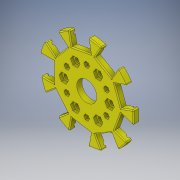
# Autodesk Inventor part: Frame
Saved by Autodesk Inventor 2016 (Build 200138000, 138)
## iProperties
Created: 2016-12-01
Part Number: Frame
Material: Generic
Document SubType Name: Modeling
Designer: Evan Phil George
Density: 1 g/cm^3
Appearance: Default
Author: Evan Phil George
Autodesk Inventor part; units mm, degrees
ref_plane "YZ Plane" through (0, 0, 0) normal (1, 0, 0) x (0, 1, 0)
ref_plane "XZ Plane" through (0, 0, 0) normal (0, 1, 0) x (-1, 0, 0)
ref_plane "XY Plane" through (0, 0, 0) normal (0, 0, 1) x (1, 0, 0)
sketch "Sketch1" plane through (0, 0, 0) normal (0, 0, 1) x (1, 0, 0)
  line L0 (0, 0) -> (49, 0)
  line L1 (0, 0) -> (-44.35, 0)
  line L2 (-44.35, 0) -> (-44.35, 10)
  line L3 (-44.35, 0) -> (-44.35, -10)
  line L4 (-44.35, 10) -> (-47.9687, 10)
  line L5 (-44.35, -10) -> (-47.9687, -10)
  line L6 (-44.35, 10) -> (-34.35, 10)
  line L7 (-34.35, 10) -> (-34.35, -10)
  line L8 (-34.35, -10) -> (-44.35, -10)
  line L9 (0, 0) -> (41.6754, 15.1686)
  line L10 (0, 0) -> (44.35, 0) construction
  line L11 (41.6754, 15.1686) -> (38.2552, 24.5655)
  line L12 (41.6754, 15.1686) -> (45.0956, 5.7717)
  line L13 (0, 0) -> (22.175, 38.4082)
  line L14 (0, 0) -> (44.35, 0) construction
  line L15 (22.175, 38.4082) -> (30.8353, 33.4082)
  line L16 (22.175, 38.4082) -> (13.5147, 43.4082)
  line L17 (0, 0) -> (-7.7013, 43.6762)
  line L18 (0, 0) -> (44.35, 0) construction
  line L19 (-7.7013, 43.6762) -> (2.1468, 45.4127)
  line L20 (-7.7013, 43.6762) -> (-17.5494, 41.9397)
  line L21 (0, 0) -> (-33.9741, 28.5076)
  line L22 (0, 0) -> (44.35, 0) construction
  line L23 (-33.9741, 28.5076) -> (-27.5462, 36.1681)
  line L24 (-33.9741, 28.5076) -> (-40.4019, 20.8472)
  line L25 (0, 0) -> (41.6754, -15.1686)
  line L26 (0, 0) -> (44.35, 0) construction
  line L27 (41.6754, -15.1686) -> (45.0956, -5.7717)
  line L28 (41.6754, -15.1686) -> (38.2552, -24.5655)
  line L29 (0, 0) -> (22.175, -38.4082)
  line L30 (0, 0) -> (44.35, 0) construction
  line L31 (22.175, -38.4082) -> (30.8353, -33.4082)
  line L32 (22.175, -38.4082) -> (13.5147, -43.4082)
  line L33 (0, 0) -> (-7.7013, -43.6762)
  line L34 (0, 0) -> (44.35, 0) construction
  line L35 (-7.7013, -43.6762) -> (2.1468, -45.4127)
  line L36 (-7.7013, -43.6762) -> (-17.5494, -41.9397)
  line L37 (0, 0) -> (-33.9741, -28.5076)
  line L38 (0, 0) -> (44.35, 0) construction
  line L39 (-33.9741, -28.5076) -> (-27.5462, -36.1681)
  line L40 (-33.9741, -28.5076) -> (-40.4019, -20.8472)
  line L41 (-27.5462, 36.1681) -> (-30.3183, 38.4942)
  line L42 (-40.4019, 20.8472) -> (-43.1741, 23.1733)
  line L43 (-27.5462, 36.1681) -> (-19.8858, 29.7402)
  line L44 (-40.4019, 20.8472) -> (-32.7415, 14.4193)
  line L45 (-17.5494, 41.9397) -> (-18.1778, 45.5035)
  line L46 (2.1468, 45.4127) -> (1.5184, 48.9765)
  line L47 (2.1468, 45.4127) -> (3.8833, 35.5646)
  line L48 (-17.5494, 41.9397) -> (-15.8129, 32.0917)
  line L49 (30.8353, 33.4082) -> (32.6446, 36.5421)
  line L50 (30.8353, 33.4082) -> (25.8353, 24.748)
  line L51 (13.5147, 43.4082) -> (15.3241, 46.5421)
  line L52 (13.5147, 43.4082) -> (8.5147, 34.748)
  line L53 (38.2552, 24.5655) -> (41.6557, 25.8032)
  line L54 (45.0956, 5.7717) -> (48.4961, 7.0093)
  line L55 (45.0956, 5.7717) -> (35.6986, 2.3515)
  line L56 (38.2552, 24.5655) -> (28.8582, 21.1453)
  line L57 (45.0956, -5.7717) -> (48.4961, -7.0093)
  line L58 (45.0956, -5.7717) -> (35.6986, -2.3515)
  line L59 (38.2552, -24.5655) -> (41.6557, -25.8032)
  line L60 (38.2552, -24.5655) -> (28.8582, -21.1453)
  line L61 (30.8353, -33.4082) -> (32.6446, -36.5421)
  line L62 (13.5147, -43.4082) -> (15.3241, -46.5421)
  line L63 (30.8353, -33.4082) -> (25.8353, -24.748)
  line L64 (13.5147, -43.4082) -> (8.5147, -34.748)
  line L65 (2.1468, -45.4127) -> (1.5184, -48.9765)
  line L66 (2.1468, -45.4127) -> (3.8833, -35.5646)
  line L67 (-17.5494, -41.9397) -> (-15.8129, -32.0917)
  line L68 (-27.5462, -36.1681) -> (-30.3183, -38.4942)
  line L69 (-40.4019, -20.8472) -> (-43.1741, -23.1733)
  line L70 (-27.5462, -36.1681) -> (-19.8858, -29.7402)
  line L71 (-40.4019, -20.8472) -> (-32.7415, -14.4193)
  line L72 (-17.5494, -41.9397) -> (-18.1778, -45.5035)
  line L73 (-32.7415, 14.4193) -> (-19.8858, 29.7402)
  line L74 (-15.8129, 32.0917) -> (3.8833, 35.5646)
  line L75 (8.5147, 34.748) -> (25.8353, 24.748)
  line L76 (28.8582, 21.1453) -> (35.6986, 2.3515)
  line L77 (35.6986, -2.3515) -> (28.8582, -21.1453)
  line L78 (25.8353, -24.748) -> (8.5147, -34.748)
  line L79 (3.8833, -35.5646) -> (-15.8129, -32.0917)
  line L80 (-19.8858, -29.7402) -> (-32.7415, -14.4193)
  arc A0 (15.3241, 46.5421) -> (1.5184, 48.9765) centre (0, 0) ccw
  arc A1 (41.6557, 25.8032) -> (32.6446, 36.5421) centre (0, 0) ccw
  arc A2 (48.4961, -7.0093) -> (48.4961, 7.0093) centre (0, 0) ccw
  arc A3 (32.6446, -36.5421) -> (41.6557, -25.8032) centre (0, 0) ccw
  arc A4 (1.5184, -48.9765) -> (15.3241, -46.5421) centre (0, 0) ccw
  arc A5 (-30.3183, -38.4942) -> (-18.1778, -45.5035) centre (0, 0) ccw
  arc A6 (-47.9687, -10) -> (-43.1741, -23.1733) centre (0, 0) ccw
  arc A7 (-18.1778, 45.5035) -> (-30.3183, 38.4942) centre (0, 0) ccw
  arc A8 (-43.1741, 23.1733) -> (-47.9687, 10) centre (0, 0) ccw
  dimension "d13" = 44.35
  dimension "d14" = 10
  dimension "d16" = 10
  dimension "d17" = 10
  dimension "d19" = 44.35
  dimension "d20" = 20
  dimension "d21" = 10
  dimension "d22" = 10
  dimension "d23" = 44.35
  dimension "d24" = 60
  dimension "d25" = 10
  dimension "d26" = 10
  dimension "d27" = 44.35
  dimension "d28" = 100
  dimension "d29" = 10
  dimension "d30" = 10
  dimension "d31" = 44.35
  dimension "d32" = 140
  dimension "d33" = 10
  dimension "d34" = 10
  dimension "d35" = 44.35
  dimension "d36" = 20
  dimension "d37" = 10
  dimension "d38" = 10
  dimension "d39" = 44.35
  dimension "d40" = 60
  dimension "d41" = 10
  dimension "d42" = 10
  dimension "d43" = 44.35
  dimension "d44" = 100
  dimension "d45" = 10
  dimension "d46" = 10
  dimension "d47" = 44.35
  dimension "d48" = 140
  dimension "d49" = 10
  dimension "d50" = 10
  dimension "d51" = 10
  dimension "d52" = 10
  dimension "d53" = 10
  dimension "d54" = 10
  dimension "d55" = 10
  dimension "d56" = 10
  dimension "d57" = 10
  dimension "d58" = 10
  dimension "d59" = 10
  dimension "d60" = 10
  dimension "d61" = 10
  dimension "d62" = 10
  dimension "d63" = 10
  dimension "d64" = 10
  dimension "d65" = 10
  dimension "d66" = 10
  constraints: 162 end point, 50 perpendicular, 19 point on circle, 13 horizontal, 9 centre point, 8 equal length, 2 vertical, 1 coincident
  measures "d13" distance of L0.start L1.end
  measures "d14" distance of L1.end L2.end
  measures "d16" distance of L1.end L3.end
  measures "d17" distance of L2.end L6.end
  measures "d19" distance of L0.start L9.end
  measures "d20" angle of L10 L9
  measures "d21" distance of L9.end L11.end
  measures "d22" distance of L9.end L12.end
  measures "d23" distance of L0.start L13.end
  measures "d24" angle of L14 L13
  measures "d25" distance of L13.end L15.end
  measures "d26" distance of L13.end L16.end
  measures "d27" distance of L0.start L17.end
  measures "d28" angle of L18 L17
  measures "d29" distance of L17.end L19.end
  measures "d30" distance of L17.end L20.end
  measures "d31" distance of L0.start L21.end
  measures "d32" angle of L22 L21
  measures "d33" distance of L21.end L23.end
  measures "d34" distance of L21.end L24.end
  measures "d35" distance of L0.start L25.end
  measures "d36" angle of L25 L26
  measures "d37" distance of L25.end L27.end
  measures "d38" distance of L25.end L28.end
  measures "d39" distance of L0.start L29.end
  measures "d40" angle of L29 L30
  measures "d41" distance of L29.end L31.end
  measures "d42" distance of L29.end L32.end
  measures "d43" distance of L0.start L33.end
  measures "d44" angle of L33 L34
  measures "d45" distance of L33.end L35.end
  measures "d46" distance of L33.end L36.end
  measures "d47" distance of L0.start L37.end
  measures "d48" angle of L37 L38
  measures "d49" distance of L37.end L39.end
  measures "d50" distance of L37.end L40.end
  measures "d51" distance of L23.end L43.end
  measures "d52" distance of L24.end L44.end
  measures "d53" distance of L19.end L47.end
  measures "d54" distance of L20.end L48.end
  measures "d55" distance of L15.end L50.end
  measures "d56" distance of L16.end L52.end
  measures "d57" distance of L12.end L55.end
  measures "d58" distance of L11.end L56.end
  measures "d59" distance of L27.end L58.end
  measures "d60" distance of L28.end L60.end
  measures "d61" distance of L31.end L63.end
  measures "d62" distance of L32.end L64.end
  measures "d63" distance of L35.end L66.end
  measures "d64" distance of L36.end L67.end
  measures "d65" distance of L39.end L70.end
  measures "d66" distance of L40.end L71.end
extrude "Extrusion1" add sketch "Sketch1" along normal blind 5.5 contours L9 L76 L55 L54 A2 L0 | L37 L80 L71 L69 A6 L5 L8 L7 L1 | L13 L75 L50 L49 A1 L53 L56 L76 L9 | L17 L74 L47 L46 A0 L51 L52 L75 L13 | L21 L73 L43 L41 A7 L45 L48 L74 L17 | L1 L7 L6 L4 A8 L42 L44 L73 L21 | L0 A2 L57 L58 L77 L25 | L25 L77 L60 L59 A3 L61 L63 L78 L29 | L29 L78 L64 L62 A4 L65 L66 L79 L33 | L33 L79 L67 L72 A5 L68 L70 L80 L37
sketch "Sketch2" plane through (15.3241, 46.5421, 5.5) normal (0.866, -0.5, 0) x (0, 0, -1)
  line L0 (5.5, -13.6187) -> (5.5, 0) projected
  circle A0 centre (5.5, -4) radius 1.55
  line L1 (5.5, 0) -> (0, 0) projected
  point P0 (5.5, -47.9687)
  dimension "d69" = 3.1
  dimension "d70" = 4
  constraints: 1 centre point, 1 point on line
  measures "d69" diameter of A0
  measures "d70" distance from line of A0.centre L1
extrude "Extrusion2" cut sketch "Sketch2" against normal blind 2
sketch "Sketch3" plane through (25.8353, 24.748, 0) normal (-0.866, 0.5, 0) x (0, 0, 1)
  line L0 (0, 13.6187) -> (0, 0) projected
  circle A0 centre (0, 9.6187) radius 1.55
  line L1 (0, 13.6187) -> (5.5, 13.6187) projected
  point P0 (0, -34.35)
  dimension "d73" = 3.1
  dimension "d74" = 4
  constraints: 1 centre point, 1 point on line
  measures "d73" diameter of A0
  measures "d74" distance from line of A0.centre L1
extrude "Extrusion3" cut sketch "Sketch3" against normal blind 2
sketch "Sketch4" plane through (41.6557, 25.8032, 0) normal (0.342, -0.9397, 0) x (0.9397, 0.342, 0)
  line L0 (-13.6187, 0) -> (0, 0) projected
  circle A0 centre (-4, 0) radius 1.55
  line L1 (0, 0) -> (0, 5.5) projected
  point P0 (-47.9687, 0)
  dimension "d77" = 3.1
  dimension "d78" = 4
  constraints: 1 centre point, 1 point on line
  measures "d77" diameter of A0
  measures "d78" distance from line of A0.centre L1
extrude "Extrusion4" cut sketch "Sketch4" against normal blind 2
sketch "Sketch5" plane through (35.6986, 2.3515, 5.5) normal (-0.342, 0.9397, 0) x (0.9397, 0.342, 0)
  line L0 (13.6187, 5.5) -> (0, 5.5) projected
  circle A0 centre (9.6187, 5.5) radius 1.55
  line L1 (13.6187, 5.5) -> (13.6187, 0) projected
  point P0 (-34.35, 5.5)
  dimension "d82" = 3.1
  dimension "d83" = 4
  constraints: 1 centre point, 1 point on line
  measures "d82" diameter of A0
  measures "d83" distance from line of A0.centre L1
extrude "Extrusion5" cut sketch "Sketch5" against normal blind 2
sketch "Sketch6" plane through (48.4961, -7.0093, 0) normal (-0.342, -0.9397, 0) x (0.9397, -0.342, 0)
  line L0 (-13.6187, 0) -> (0, 0) projected
  circle A0 centre (-4, 0) radius 1.55
  line L1 (0, 0) -> (0, 5.5) projected
  point P0 (-47.9687, 0)
  dimension "d86" = 3.1
  dimension "d87" = 4
  constraints: 1 centre point, 1 point on line
  measures "d86" diameter of A0
  measures "d87" distance from line of A0.centre L1
extrude "Extrusion6" cut sketch "Sketch6" against normal blind 2
sketch "Sketch7" plane through (28.8582, -21.1453, 5.5) normal (0.342, 0.9397, 0) x (0.9397, -0.342, 0)
  line L0 (13.6187, 5.5) -> (0, 5.5) projected
  circle A0 centre (9.6187, 5.5) radius 1.55
  line L1 (13.6187, 5.5) -> (13.6187, 0) projected
  point P0 (-34.35, 5.5)
  dimension "d90" = 3.1
  dimension "d91" = 4
  constraints: 1 centre point, 1 point on line
  measures "d90" diameter of A0
  measures "d91" distance from line of A0.centre L1
extrude "Extrusion7" cut sketch "Sketch7" against normal blind 2
sketch "Sketch8" plane through (32.6446, -36.5421, 0) normal (-0.866, -0.5, 0) x (0, 0, 1)
  line L0 (0, 13.6187) -> (0, 0) projected
  circle A0 centre (0, 4) radius 1.55
  line L1 (0, 0) -> (5.5, 0) projected
  point P0 (0, 47.9687)
  dimension "d94" = 3.1
  dimension "d95" = 4
  constraints: 1 centre point, 1 point on line
  measures "d94" diameter of A0
  measures "d95" distance from line of A0.centre L1
extrude "Extrusion8" cut sketch "Sketch8" against normal blind 2
sketch "Sketch9" plane through (8.5147, -34.748, 5.5) normal (0.866, 0.5, 0) x (0, 0, -1)
  line L0 (5.5, -13.6187) -> (5.5, 0) projected
  circle A0 centre (5.5, -9.6187) radius 1.55
  line L1 (5.5, -13.6187) -> (0, -13.6187) projected
  point P0 (5.5, 34.35)
  dimension "d98" = 3.1
  dimension "d99" = 4
  constraints: 1 centre point, 1 point on line
  measures "d98" diameter of A0
  measures "d99" distance from line of A0.centre L1
extrude "Extrusion9" cut sketch "Sketch9" against normal blind 2
sketch "Sketch10" plane through (1.5184, -48.9765, 0) normal (-0.9848, 0.1736, 0) x (0, 0, 1)
  line L0 (0, 13.6187) -> (0, 0) projected
  circle A0 centre (0, 4) radius 1.55
  line L1 (0, 0) -> (5.5, 0) projected
  point P0 (0, 47.9687)
  dimension "d102" = 3.1
  dimension "d103" = 4
  constraints: 1 centre point, 1 point on line
  measures "d102" diameter of A0
  measures "d103" distance from line of A0.centre L1
extrude "Extrusion10" cut sketch "Sketch10" against normal blind 2
sketch "Sketch11" plane through (-15.8129, -32.0917, 5.5) normal (0.9848, -0.1736, 0) x (0, 0, -1)
  line L0 (5.5, -13.6187) -> (5.5, 0) projected
  circle A0 centre (5.5, -9.6187) radius 1.55
  line L1 (5.5, -13.6187) -> (0, -13.6187) projected
  point P0 (5.5, 34.35)
  dimension "d106" = 3.1
  dimension "d107" = 4
  constraints: 1 centre point, 1 point on line
  measures "d106" diameter of A0
  measures "d107" distance from line of A0.centre L1
extrude "Extrusion11" cut sketch "Sketch11" against normal blind 2
sketch "Sketch12" plane through (-30.3183, -38.4942, 5.5) normal (-0.6428, 0.766, 0) x (0.766, 0.6428, 0)
  line L0 (13.6187, 5.5) -> (0, 5.5) projected
  circle A0 centre (4, 5.5) radius 1.55
  line L1 (0, 5.5) -> (0, 0) projected
  point P0 (47.9687, 5.5)
  dimension "d110" = 3.1
  dimension "d111" = 4
  constraints: 1 centre point, 1 point on line
  measures "d110" diameter of A0
  measures "d111" distance from line of A0.centre L1
extrude "Extrusion12" cut sketch "Sketch12" against normal blind 2
sketch "Sketch13" plane through (-32.7415, -14.4193, 0) normal (0.6428, -0.766, 0) x (0.766, 0.6428, 0)
  line L0 (-13.6187, 0) -> (0, 0) projected
  circle A0 centre (-9.6187, 0) radius 1.55
  line L1 (-13.6187, 0) -> (-13.6187, 5.5) projected
  point P0 (34.35, 0)
  dimension "d114" = 3.1
  dimension "d115" = 4
  constraints: 1 centre point, 1 point on line
  measures "d114" diameter of A0
  measures "d115" distance from line of A0.centre L1
extrude "Extrusion13" cut sketch "Sketch13" against normal blind 2
sketch "Sketch14" plane through (-47.9687, -10, 0) normal (0, 1, 0) x (1, 0, 0)
  line L0 (13.6187, 0) -> (0, 0) projected
  circle A0 centre (4, 0) radius 1.55
  line L1 (0, 0) -> (0, -5.5) projected
  point P0 (47.9687, 0)
  dimension "d118" = 3.1
  dimension "d119" = 4
  constraints: 1 centre point, 1 point on line
  measures "d118" diameter of A0
  measures "d119" distance from line of A0.centre L1
extrude "Extrusion14" cut sketch "Sketch14" against normal blind 2
sketch "Sketch15" plane through (-47.9687, 10, 0) normal (0, -1, 0) x (1, 0, 0)
  line L0 (0, 0) -> (13.6187, 0) projected
  circle A0 centre (4, 0) radius 1.55
  line L1 (0, 0) -> (0, 5.5) projected
  point P0 (47.9687, 0)
  dimension "d122" = 3.1
  dimension "d123" = 4
  constraints: 1 centre point, 1 point on line
  measures "d122" diameter of A0
  measures "d123" distance from line of A0.centre L1
extrude "Extrusion15" cut sketch "Sketch15" against normal blind 2
sketch "Sketch16" plane through (-43.1741, 23.1733, 5.5) normal (0.6428, 0.766, 0) x (0.766, -0.6428, 0)
  line L0 (13.6187, 5.5) -> (0, 5.5) projected
  circle A0 centre (4, 5.5) radius 1.55
  line L1 (0, 5.5) -> (0, 0) projected
  point P0 (47.9687, 5.5)
  dimension "d126" = 3.1
  dimension "d127" = 4
  constraints: 1 centre point, 1 point on line
  measures "d126" diameter of A0
  measures "d127" distance from line of A0.centre L1
extrude "Extrusion16" cut sketch "Sketch16" against normal blind 2
sketch "Sketch17" plane through (-19.8858, 29.7402, 0) normal (-0.6428, -0.766, 0) x (0.766, -0.6428, 0)
  line L0 (-13.6187, 0) -> (0, 0) projected
  circle A0 centre (-9.6187, 0) radius 1.55
  line L1 (-13.6187, 0) -> (-13.6187, 5.5) projected
  point P0 (34.35, 0)
  dimension "d130" = 3.1
  dimension "d131" = 4
  constraints: 1 centre point, 1 point on line
  measures "d130" diameter of A0
  measures "d131" distance from line of A0.centre L1
extrude "Extrusion17" cut sketch "Sketch17" against normal blind 2
sketch "Sketch18" plane through (-18.1778, 45.5035, 5.5) normal (0.9848, 0.1736, 0) x (0, 0, -1)
  line L0 (5.5, -13.6187) -> (5.5, 0) projected
  circle A0 centre (5.5, -4) radius 1.55
  line L1 (5.5, 0) -> (0, 0) projected
  point P0 (5.5, -47.9687)
  dimension "d134" = 3.1
  dimension "d135" = 4
  constraints: 1 centre point, 1 point on line
  measures "d134" diameter of A0
  measures "d135" distance from line of A0.centre L1
extrude "Extrusion18" cut sketch "Sketch18" against normal blind 2
sketch "Sketch19" plane through (3.8833, 35.5646, 0) normal (-0.9848, -0.1736, 0) x (0, 0, 1)
  line L0 (0, 13.6187) -> (0, 0) projected
  circle A0 centre (0, 9.6187) radius 1.55
  line L1 (0, 13.6187) -> (5.5, 13.6187) projected
  point P0 (0, -34.35)
  dimension "d138" = 3.1
  dimension "d139" = 4
  constraints: 1 centre point, 1 point on line
  measures "d138" diameter of A0
  measures "d139" distance from line of A0.centre L1
extrude "Extrusion19" cut sketch "Sketch19" against normal blind 2
sketch "Sketch20" plane through (0, 0, 5.5) normal (0, 0, 1) x (1, 0, 0)
  line L0 (0, 0) -> (23.85, 0)
  line L1 (0, 0) -> (11.925, 20.6547)
  line L2 (0, 0) -> (23.85, 0) construction
  line L3 (0, 0) -> (-11.925, 20.6547)
  line L4 (0, 0) -> (23.85, 0) construction
  line L5 (0, 0) -> (-23.85, 0)
  line L6 (0, 0) -> (11.925, -20.6547)
  line L7 (0, 0) -> (23.85, 0) construction
  line L8 (0, 0) -> (-11.925, -20.6547)
  line L9 (0, 0) -> (23.85, 0) construction
  line L10 (0, 0) -> (20.6547, 11.925)
  line L11 (0, 0) -> (23.85, 0) construction
  line L12 (0, 0) -> (0, 23.85)
  line L13 (0, 0) -> (23.85, 0) construction
  line L14 (0, 0) -> (-20.6547, 11.925)
  line L15 (0, 0) -> (23.85, 0) construction
  line L16 (0, 0) -> (20.6547, -11.925)
  line L17 (0, 0) -> (23.85, 0) construction
  line L18 (0, 0) -> (0, -23.85)
  line L19 (0, 0) -> (23.85, 0) construction
  line L20 (0, 0) -> (-20.6547, -11.925)
  line L21 (0, 0) -> (23.85, 0) construction
  line L22 (28.85, 0) -> (26.35, -4.3301)
  line L23 (26.35, -4.3301) -> (21.35, -4.3301)
  line L24 (21.35, -4.3301) -> (18.85, 0)
  line L25 (18.85, 0) -> (21.35, 4.3301)
  line L26 (21.35, 4.3301) -> (26.35, 4.3301)
  line L27 (26.35, 4.3301) -> (28.85, 0)
  line L28 (23.6547, 11.925) -> (22.1547, 9.3269)
  line L29 (22.1547, 9.3269) -> (19.1547, 9.3269)
  line L30 (19.1547, 9.3269) -> (17.6547, 11.925)
  line L31 (17.6547, 11.925) -> (19.1547, 14.5231)
  line L32 (19.1547, 14.5231) -> (22.1547, 14.5231)
  line L33 (22.1547, 14.5231) -> (23.6547, 11.925)
  line L34 (-6.925, 20.6547) -> (-9.425, 16.3246)
  line L35 (-9.425, 16.3246) -> (-14.425, 16.3246)
  line L36 (-14.425, 16.3246) -> (-16.925, 20.6547)
  line L37 (-16.925, 20.6547) -> (-14.425, 24.9848)
  line L38 (-14.425, 24.9848) -> (-9.425, 24.9848)
  line L39 (-9.425, 24.9848) -> (-6.925, 20.6547)
  line L40 (-23.6547, 11.925) -> (-22.1547, 14.5231)
  line L41 (-22.1547, 14.5231) -> (-19.1547, 14.5231)
  line L42 (-19.1547, 14.5231) -> (-17.6547, 11.925)
  line L43 (-17.6547, 11.925) -> (-19.1547, 9.3269)
  line L44 (-19.1547, 9.3269) -> (-22.1547, 9.3269)
  line L45 (-22.1547, 9.3269) -> (-23.6547, 11.925)
  line L46 (-28.85, 0) -> (-26.35, 4.3301)
  line L47 (-26.35, 4.3301) -> (-21.35, 4.3301)
  line L48 (-21.35, 4.3301) -> (-18.85, 0)
  line L49 (-18.85, 0) -> (-21.35, -4.3301)
  line L50 (-21.35, -4.3301) -> (-26.35, -4.3301)
  line L51 (-26.35, -4.3301) -> (-28.85, 0)
  line L52 (-23.6546, -11.9058) -> (-22.138, -9.3174)
  line L53 (-22.138, -9.3174) -> (-19.1381, -9.3366)
  line L54 (-19.1381, -9.3366) -> (-17.6548, -11.9442)
  line L55 (-17.6548, -11.9442) -> (-19.1714, -14.5326)
  line L56 (-19.1714, -14.5326) -> (-22.1713, -14.5134)
  line L57 (-22.1713, -14.5134) -> (-23.6546, -11.9058)
  line L58 (-16.925, -20.6547) -> (-14.425, -16.3246)
  line L59 (-14.425, -16.3246) -> (-9.425, -16.3246)
  line L60 (-9.425, -16.3246) -> (-6.925, -20.6547)
  line L61 (-6.925, -20.6547) -> (-9.425, -24.9848)
  line L62 (-9.425, -24.9848) -> (-14.425, -24.9848)
  line L63 (-14.425, -24.9848) -> (-16.925, -20.6547)
  line L64 (3, -23.85) -> (1.5, -26.4481)
  line L65 (1.5, -26.4481) -> (-1.5, -26.4481)
  line L66 (-1.5, -26.4481) -> (-3, -23.85)
  line L67 (-3, -23.85) -> (-1.5, -21.2519)
  line L68 (-1.5, -21.2519) -> (1.5, -21.2519)
  line L69 (1.5, -21.2519) -> (3, -23.85)
  line L70 (16.925, -20.6547) -> (14.425, -24.9848)
  line L71 (14.425, -24.9848) -> (9.425, -24.9848)
  line L72 (9.425, -24.9848) -> (6.925, -20.6547)
  line L73 (6.925, -20.6547) -> (9.425, -16.3246)
  line L74 (9.425, -16.3246) -> (14.425, -16.3246)
  line L75 (14.425, -16.3246) -> (16.925, -20.6547)
  line L76 (23.6547, -11.9108) -> (22.167, -14.516)
  line L77 (22.167, -14.516) -> (19.167, -14.5302)
  line L78 (19.167, -14.5302) -> (17.6547, -11.9392)
  line L79 (17.6547, -11.9392) -> (19.1425, -9.334)
  line L80 (19.1425, -9.334) -> (22.1425, -9.3198)
  line L81 (22.1425, -9.3198) -> (23.6547, -11.9108)
  line L82 (-3, 23.85) -> (-1.5, 26.4481)
  line L83 (-1.5, 26.4481) -> (1.5, 26.4481)
  line L84 (1.5, 26.4481) -> (3, 23.85)
  line L85 (3, 23.85) -> (1.5, 21.2519)
  line L86 (1.5, 21.2519) -> (-1.5, 21.2519)
  line L87 (-1.5, 21.2519) -> (-3, 23.85)
  line L88 (16.925, 20.6547) -> (14.425, 16.3246)
  line L89 (14.425, 16.3246) -> (9.425, 16.3246)
  line L90 (9.425, 16.3246) -> (6.925, 20.6547)
  line L91 (6.925, 20.6547) -> (9.425, 24.9848)
  line L92 (9.425, 24.9848) -> (14.425, 24.9848)
  line L93 (14.425, 24.9848) -> (16.925, 20.6547)
  dimension "d142" = 23.85
  dimension "d143" = 23.85
  dimension "d144" = 60
  dimension "d145" = 23.85
  dimension "d146" = 120
  dimension "d147" = 23.85
  dimension "d148" = 23.85
  dimension "d149" = 60
  dimension "d150" = 23.85
  dimension "d151" = 120
  dimension "d152" = 23.85
  dimension "d153" = 30
  dimension "d154" = 23.85
  dimension "d155" = 90
  dimension "d156" = 23.85
  dimension "d157" = 150
  dimension "d158" = 23.85
  dimension "d159" = 30
  dimension "d160" = 23.85
  dimension "d161" = 90
  dimension "d162" = 23.85
  dimension "d163" = 150
  dimension "d164" = 5
  dimension "d165" = 3
  dimension "d168" = 5
  dimension "d169" = 3
  dimension "d170" = 5
  dimension "d171" = 3
  dimension "d172" = 5
  dimension "d173" = 3
  dimension "d174" = 5
  dimension "d176" = 3
  dimension "d177" = 3
  dimension "d178" = 5
  constraints: 188 end point, 12 coincident, 11 horizontal, 10 equal length, 2 perpendicular, 1 point on line, 1 vertical, 156 other
  measures "d142" distance of L0.start L0.end
  measures "d143" distance of L0.start L1.end
  measures "d144" angle of L2 L1
  measures "d145" distance of L0.start L3.end
  measures "d146" angle of L4 L3
  measures "d147" distance of L0.start L5.end
  measures "d148" distance of L0.start L6.end
  measures "d149" angle of L6 L7
  measures "d150" distance of L0.start L8.end
  measures "d151" angle of L8 L9
  measures "d152" distance of L0.start L10.end
  measures "d153" angle of L11 L10
  measures "d154" distance of L0.start L12.end
  measures "d155" angle of L13 L12
  measures "d156" distance of L0.start L14.end
  measures "d157" angle of L15 L14
  measures "d158" distance of L0.start L16.end
  measures "d159" angle of L16 L17
  measures "d160" distance of L0.start L18.end
  measures "d161" angle of L18 L19
  measures "d162" distance of L0.start L20.end
  measures "d163" angle of L20 L21
  measures "d164" distance of L25.end L26.end
  measures "d165" distance of L31.end L32.end
  measures "d168" distance of L37.end L38.end
  measures "d169" distance of L40.end L41.end
  measures "d170" distance of L46.end L47.end
  measures "d171" distance of L55.end L56.end
  measures "d172" distance of L58.end L59.end
  measures "d173" distance of L67.end L68.end
  measures "d174" distance of L73.end L74.end
  measures "d176" horizontal distance of L79.end L80.end
  measures "d177" distance of L82.end L83.end
  measures "d178" distance of L91.end L92.end
extrude "Extrusion20" cut sketch "Sketch20" against normal blind 2.75
sketch "Sketch21" plane through (0, 0, 0) normal (0, 0, -1) x (-1, 0, 0)
  line L0 (0, 0) -> (20.6547, 11.925)
  line L1 (0, 0) -> (23.85, 0) construction
  line L2 (0, 0) -> (11.925, 20.6547)
  line L3 (0, 0) -> (23.85, 0) construction
  line L4 (0, 0) -> (0, 23.85)
  line L5 (0, 0) -> (23.85, 0) construction
  line L6 (0, 0) -> (-11.925, 20.6547)
  line L7 (0, 0) -> (23.85, 0) construction
  line L8 (0, 0) -> (-20.6547, 11.925)
  line L9 (0, 0) -> (23.85, 0) construction
  line L10 (0, 0) -> (-23.85, 0)
  line L11 (0, 0) -> (23.85, 0) construction
  line L12 (0, 0) -> (23.85, 0)
  line L13 (0, 0) -> (20.6547, -11.925)
  line L14 (0, 0) -> (23.85, 0) construction
  line L15 (0, 0) -> (11.925, -20.6547)
  line L16 (0, 0) -> (23.85, 0) construction
  line L17 (0, 0) -> (0, -23.85)
  line L18 (0, 0) -> (23.85, 0) construction
  line L19 (0, 0) -> (-11.925, -20.6547)
  line L20 (0, 0) -> (23.85, 0) construction
  line L21 (0, 0) -> (-20.6547, -11.925)
  line L22 (0, 0) -> (23.85, 0) construction
  circle A0 centre (23.85, 0) radius 2.5
  circle A1 centre (20.6547, 11.925) radius 1.5
  circle A2 centre (11.925, 20.6547) radius 2.5
  circle A3 centre (0, 23.85) radius 1.5
  circle A4 centre (-11.925, 20.6547) radius 2.5
  circle A5 centre (-20.6547, 11.925) radius 1.5
  circle A6 centre (-23.85, 0) radius 2.5
  circle A7 centre (-20.6547, -11.925) radius 1.5
  circle A8 centre (-11.925, -20.6547) radius 2.5
  circle A9 centre (0, -23.85) radius 1.5
  circle A10 centre (11.925, -20.6547) radius 2.5
  circle A11 centre (20.6547, -11.925) radius 1.5
  dimension "d181" = 23.85
  dimension "d182" = 30
  dimension "d183" = 23.85
  dimension "d184" = 60
  dimension "d185" = 23.85
  dimension "d186" = 90
  dimension "d187" = 23.85
  dimension "d188" = 120
  dimension "d189" = 23.85
  dimension "d190" = 150
  dimension "d191" = 23.85
  dimension "d192" = 180
  dimension "d193" = 23.85
  dimension "d194" = 23.85
  dimension "d195" = 30
  dimension "d196" = 23.85
  dimension "d197" = 60
  dimension "d198" = 23.85
  dimension "d199" = 90
  dimension "d200" = 23.85
  dimension "d201" = 120
  dimension "d202" = 23.85
  dimension "d203" = 150
  dimension "d204" = 5
  dimension "d205" = 3
  dimension "d206" = 5
  dimension "d207" = 3
  dimension "d208" = 5
  dimension "d209" = 3
  dimension "d210" = 5
  dimension "d211" = 3
  dimension "d212" = 5
  dimension "d213" = 3
  dimension "d214" = 5
  dimension "d215" = 3
  constraints: 46 end point, 12 centre point, 12 coincident, 12 horizontal, 11 equal length, 2 perpendicular, 1 collinear, 1 vertical
  measures "d181" distance of L0.start L0.end
  measures "d182" angle of L1 L0
  measures "d183" distance of L0.start L2.end
  measures "d184" angle of L3 L2
  measures "d185" distance of L0.start L4.end
  measures "d186" angle of L5 L4
  measures "d187" distance of L0.start L6.end
  measures "d188" angle of L7 L6
  measures "d189" distance of L0.start L8.end
  measures "d190" angle of L9 L8
  measures "d191" distance of L0.start L10.end
  measures "d192" angle of L10 L11
  measures "d193" distance of L0.start L11.end
  measures "d194" distance of L0.start L13.end
  measures "d195" angle of L13 L14
  measures "d196" distance of L0.start L15.end
  measures "d197" angle of L15 L16
  measures "d198" distance of L0.start L17.end
  measures "d199" angle of L17 L18
  measures "d200" distance of L0.start L19.end
  measures "d201" angle of L19 L20
  measures "d202" distance of L0.start L21.end
  measures "d203" angle of L21 L22
  measures "d204" diameter of A0
  measures "d205" diameter of A1
  measures "d206" diameter of A2
  measures "d207" diameter of A3
  measures "d208" diameter of A4
  measures "d209" diameter of A5
  measures "d210" diameter of A6
  measures "d211" diameter of A7
  measures "d212" diameter of A8
  measures "d213" diameter of A9
  measures "d214" diameter of A10
  measures "d215" diameter of A11
extrude "Extrusion21" cut sketch "Sketch21" against normal blind 2.75
sketch "Sketch22" plane through (0, 0, 5.5) normal (0, 0, 1) x (1, 0, 0)
  circle A0 centre (0, 0) radius 10.5
  dimension "d218" = 21
  constraints: 1 centre point, 1 coincident
  measures "d218" diameter of A0
extrude "Extrusion22" cut sketch "Sketch22" against normal blind 5.5
fillet "Fillet1" radius 1 52 edges at (-18.1778, 45.5035, 2.75) (-24.5, 42.4352, 5.5) (-30.3183, 38.4942, 2.75) (-26.3136, 22.0798, 5.5) (-37.9578, 18.7963, 5.5) (-25.102, 34.1172, 5.5) (-16.9953, 38.7976, 5.5) (-5.9648, 33.8281, 5.5) (2.7008, 42.2705, 5.5) (1.5184, 48.9765, 2.75) (8.5088, 48.2556, 5.5) (15.3241, 46.5421, 2.75) (11.9194, 40.6451, 5.5) (17.175, 29.748, 5.5) (29.2399, 30.6451, 5.5) (32.6446, 36.5421, 2.75) (41.6557, 25.8032, 2.75) (35.257, 23.4743, 5.5) (32.2784, 11.7484, 5.5) (42.0974, 4.6804, 5.5) (48.4961, 7.0093, 2.75) (49, 0, 5.5) (48.4961, -7.0093, 2.75) (42.0974, -4.6804, 5.5) (32.2784, -11.7484, 5.5) (35.257, -23.4743, 5.5) (37.5362, -31.4966, 5.5) (41.6557, -25.8032, 2.75) (32.6446, -36.5421, 2.75) (29.2399, -30.6451, 5.5) (17.175, -29.748, 5.5) (11.9194, -40.6451, 5.5) (15.3241, -46.5421, 2.75) (8.5088, -48.2556, 5.5) (1.5184, -48.9765, 2.75) (2.7008, -42.2705, 5.5) (-5.9648, -33.8281, 5.5) (-16.9953, -38.7976, 5.5) (-18.1778, -45.5035, 2.75) (-24.5, -42.4352, 5.5) (-30.3183, -38.4942, 2.75) (-25.102, -34.1172, 5.5) (-26.3136, -22.0798, 5.5) (-37.9578, -18.7963, 5.5) (-43.1741, -23.1733, 2.75) (-46.0449, -16.759, 5.5) (-41.1594, -10, 5.5) (-47.9687, -10, 2.75) (-34.35, 0, 5.5) (-41.1594, 10, 5.5) (-47.9687, 10, 2.75) (-43.1741, 23.1733, 2.75)
body "Solid1"
